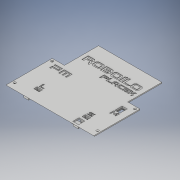
# Autodesk Inventor part: dach2
Saved by Autodesk Inventor 2019 (Build 230136000, 136)
## iProperties
Created: 2019-09-08
Part Number: dach2
Material: Generic
Document SubType Name: Modeling
Designer: Michal
Density: 1 g/cm^3
Appearance: Default
Author: Michal
Autodesk Inventor part; units mm, degrees
ref_plane "YZ Plane" through (0, 0, 0) normal (1, 0, 0) x (0, 1, 0)
ref_plane "XZ Plane" through (0, 0, 0) normal (0, 1, 0) x (-1, 0, 0)
ref_plane "XY Plane" through (0, 0, 0) normal (0, 0, 1) x (1, 0, 0)
sketch "Sketch1" plane through (0, 0, 0) normal (0, 1, 0) x (-1, 0, 0)
  line L0 (0, 0) -> (180, 0)
  line L1 (180, 0) -> (180, -95)
  line L2 (0, 0) -> (0, -95)
  line L3 (180, -95) -> (155, -95)
  line L4 (0, -95) -> (25, -95)
  line L5 (25, -95) -> (25, -165)
  line L6 (155, -95) -> (155, -165)
  line L7 (155, -165) -> (25, -165)
  dimension "d0" = 180
  dimension "d1" = 95
  dimension "d4" = 95
  dimension "d35" = 25
  dimension "d36" = 25
  constraints: 16 end point, 4 horizontal, 2 perpendicular, 2 vertical
  measures "d0" distance of L0.start L0.end
  measures "d1" distance of L0.end L1.end
  measures "d4" distance of L0.start L2.end
  measures "d35" distance of L1.end L3.end
  measures "d36" distance of L2.end L4.end
extrude "Extrusion1" add sketch "Sketch1" along normal blind 2
sketch "Sketch3" plane through (-155, 0, -165) normal (-1, 0, 0) x (0, 0, 1)
  line L0 (70, 2) -> (0, 2) projected
  line L1 (0, 2) -> (28, 2)
  line L2 (28, 2) -> (28, -13)
  circle A0 centre (28, -13) radius 12.5
  point P0 (165, 0)
  dimension "d46" = 28
  dimension "d47" = 15
  dimension "d48" = 25
  constraints: 4 end point, 1 centre point, 1 coincident, 1 perpendicular, 1 point on line
  measures "d46" distance of L0.end L1.end
  measures "d47" distance of L1.end L2.end
  measures "d48" diameter of A0
extrude "Extrusion3" cut sketch "Sketch3" against normal blind 130
chamfer "Chamfer1" distance 2 angle 45 1 edges at (-90, 0, 0)
sketch "Sketch22" plane through (0, 0, 0) normal (0, -1, 0) x (1, 0, 0)
  line L0 (0, -95.1062) -> (-10, -95.1062)
  line L1 (-10, -95.1062) -> (-10, -85.1062)
  line L2 (-10, -85.1062) -> (0, -85.1062)
  line L3 (-180, -85.1062) -> (-180, -95.1062)
  line L4 (0, -95) -> (0, -2) projected
  line L5 (0, -2) -> (-34, -2)
  line L6 (-180, -2) -> (0, -2) projected
  line L7 (-34, -2) -> (-44, -2)
  line L8 (-10, -85.1062) -> (-10, -46.6062)
  line L9 (-10, -46.6062) -> (-34, -46.6062)
  line L10 (-34, -46.6062) -> (-34, -2)
  line L11 (-10, -85.1062) -> (-25, -85.1062)
  line L12 (-25, -95) -> (-25, -165) projected
  line L13 (-44, -2) -> (-44, -46.6062)
  line L14 (-44, -46.6062) -> (-44, -56.6062)
  line L15 (-44, -56.6062) -> (-25, -56.6062)
  line L16 (-25, -56.6062) -> (-25, -85.1062)
  line L17 (-180, -95.1062) -> (-170, -95.1062)
  line L18 (-170, -95.1062) -> (-170, -85.1062)
  line L19 (-170, -85.1062) -> (-180, -85.1062)
  line L20 (-180, -2) -> (-146, -2)
  line L21 (-146, -2) -> (-136, -2)
  line L22 (-170, -85.1062) -> (-170, -46.6062)
  line L23 (-170, -46.6062) -> (-146, -46.6062)
  line L24 (-146, -46.6062) -> (-146, -2)
  line L25 (-170, -85.1062) -> (-155, -85.1062)
  line L26 (-136, -2) -> (-136, -46.6062)
  line L27 (-136, -46.6062) -> (-136, -56.6062)
  line L28 (-136, -56.6062) -> (-155, -56.6062)
  line L29 (-155, -56.6062) -> (-155, -85.1062)
  line L30 (-25, -165) -> (-38.1, -165)
  line L31 (-25, -165) -> (-155, -165) projected
  line L32 (-155, -165) -> (-155, -95) projected
  line L33 (-155, -165) -> (-141.9, -165)
  line L34 (-38.1, -165) -> (-141.9098, -165)
  line L35 (-141.9098, -165) -> (-141.9098, -113)
  line L36 (-141.9098, -113) -> (-38.1, -113)
  line L37 (-38.1, -113) -> (-38.1, -165)
  line L38 (-34, -2) -> (-34, -2.25)
  line L39 (-34, -2.25) -> (-44, -2.25)
  line L40 (-34, -2.25) -> (-34.25, -2.25)
  line L41 (-34.25, -2.25) -> (-34.25, -46.6062)
  line L42 (-34.25, -46.6062) -> (-34.25, -46.8562)
  line L43 (-34.25, -46.8562) -> (-10, -46.8562)
  line L44 (-10, -46.8562) -> (-10.25, -46.8562)
  line L45 (-10.25, -46.8562) -> (-10.25, -85.1062)
  line L46 (-10.25, -85.1062) -> (-10.25, -84.8562)
  line L47 (-10.25, -84.8562) -> (-25, -84.8562)
  line L48 (-146, -2) -> (-146, -2.25)
  line L49 (-146, -2.25) -> (-136, -2.25)
  line L50 (-146, -2.25) -> (-145.75, -2.25)
  line L51 (-145.75, -2.25) -> (-145.75, -46.6062)
  line L52 (-145.75, -46.6062) -> (-145.75, -46.8562)
  line L53 (-145.75, -46.8562) -> (-170, -46.8562)
  line L54 (-170, -46.8562) -> (-169.75, -46.8562)
  line L55 (-169.75, -85.1062) -> (-169.75, -84.8562)
  line L56 (-169.75, -84.8562) -> (-155, -84.8562)
  line L57 (-141.9098, -165) -> (-141.6598, -165)
  line L58 (-155, -165) -> (-25, -165) projected
  line L59 (-141.6598, -165) -> (-141.6598, -113)
  line L60 (-38.1, -113) -> (-38.35, -113)
  line L61 (-38.35, -113) -> (-38.35, -165)
  line L62 (-169.75, -84.8562) -> (-169.75, -46.8562)
  point P0 (0, 0)
  dimension "d215" = 10
  dimension "d216" = 10
  dimension "d217" = 34
  dimension "d218" = 10
  dimension "d219" = 38.5
  dimension "d220" = 10
  dimension "d221" = 13.1
  dimension "d222" = 13.1
  dimension "d223" = 103.8098
  dimension "d224" = 52
  dimension "d234" = 0.25
  dimension "d235" = 0.25
  dimension "d236" = 0.25
  dimension "d237" = 0.25
  dimension "d238" = 0.25
  dimension "d239" = 0.25
  dimension "d240" = 0.25
  dimension "d241" = 0.25
  dimension "d242" = 0.25
  dimension "d243" = 0.25
  dimension "d244" = 0.25
  dimension "d245" = 0.25
  constraints: 112 end point, 28 point on line, 17 perpendicular, 5 parallel, 3 vertical, 2 horizontal, 1 coincident, 4 other
  measures "d215" distance of L2.end L1.end
  measures "d216" distance of L0.end L1.end
  measures "d217" distance of L5.start L5.end
  measures "d218" distance of L5.end L7.end
  measures "d219" distance of L1.end L8.end
  measures "d220" distance of L13.end L14.end
  measures "d221" distance of L12.end L30.end
  measures "d222" distance of L31.end L33.end
  measures "d223" distance of L35.end L36.end
  measures "d224" distance of L34.end L35.end
  measures "d234" distance of L5.end L38.end
  measures "d235" distance of L38.end L40.end
  measures "d236" distance of L41.end L42.end
  measures "d237" distance of L43.end L44.end
  measures "d238" distance of L45.end L46.end
  measures "d239" distance of L20.end L48.end
  measures "d240" distance of L48.end L50.end
  measures "d241" distance of L51.end L52.end
  measures "d242" distance of L53.end L54.end
  measures "d243" distance of L55.start L55.end
  measures "d244" distance of L34.end L57.end
  measures "d245" distance of L36.end L60.end
extrude "Extrusion24" add sketch "Sketch22" along normal blind 4 contours L45 L47 L16 L15 L14 L13 L39 L41 L42 L43 | L53 L52 L51 L49 L26 L27 L28 L29 L56 L62 | L31 L61 L36 L37 | L31 L59 L36 L61 | L31 L35 L36 L59
sketch "Sketch7" plane through (0, 2, 0) normal (0, 1, 0) x (1, 0, 0)
  line L0 (-155, 95) -> (-180, 95) projected
  line L1 (-180, 95) -> (-175, 95)
  line L2 (-175, 95) -> (-175, 90)
  line L3 (-175, 90) -> (-180, 90)
  line L4 (-180, 90) -> (-180, 95)
  line L5 (0, 95) -> (-25, 95) projected
  line L6 (0, 95) -> (-5, 95)
  line L7 (-5, 95) -> (-5, 90)
  line L8 (-5, 90) -> (0, 90)
  line L9 (0, 90) -> (0, 95)
  line L10 (-5, 90) -> (-5, 13)
  line L11 (-175, 90) -> (-175, 13)
  point P0 (0, 0)
  dimension "d80" = 5
  dimension "d81" = 5
  dimension "d82" = 5
  dimension "d83" = 77
  constraints: 20 end point, 4 parallel, 2 horizontal, 2 perpendicular, 2 vertical, 1 point on line
  measures "d80" distance of L2.end L3.end
  measures "d81" distance of L1.end L2.end
  measures "d82" distance of L8.end L7.end
  measures "d83" distance of L7.end L10.end
hole "Hole1" at (-175, 2, -90) at (-5, 2, -90) at (-5, 2, -13) at (-175, 2, -13) direction (0, -1, 0) diameter 2.4638 depth 8.7884 countersink diameter 5 countersink angle 75
sketch "Sketch8" plane through (0, 2, 0) normal (0, 1, 0) x (1, 0, 0)
  line L0 (0, 0) -> (0, 95) projected
  line L1 (0, 95) -> (-13, 95)
  line L2 (-13, 95) -> (-13, 82)
  line L3 (-13, 82) -> (0, 82)
  line L4 (0, 82) -> (0, 95)
  line L5 (-13, 82) -> (-23.5, 82)
  line L6 (-23.5, 82) -> (-23.5, 67)
  line L7 (-23.5, 67) -> (-13, 67)
  line L8 (-13, 67) -> (-13, 82)
  line L9 (-180, 95) -> (-180, 0) projected
  line L10 (-180, 0) -> (0, 0) projected
  line L11 (0, 0) -> (-35, 0)
  line L12 (-35, 0) -> (-35, 4)
  line L13 (-35, 4) -> (0, 4)
  line L14 (0, 4) -> (0, 0)
  line L15 (-35, 4) -> (-47, 4)
  line L16 (-47, 4) -> (-47, 17)
  line L17 (-47, 17) -> (-35, 17)
  line L18 (-35, 17) -> (-35, 4)
  line L19 (-35, 17) -> (-35, 22)
  line L20 (-35, 22) -> (-46, 22)
  line L21 (-46, 22) -> (-46, 29)
  line L22 (-46, 29) -> (-35, 29)
  line L23 (-35, 29) -> (-35, 22)
  line L24 (-180, 0) -> (-145, 0)
  line L25 (-145, 0) -> (-145, 22)
  line L26 (-145, 22) -> (-180, 22)
  line L27 (-180, 22) -> (-180, 0)
  line L28 (-145, 22) -> (-134, 22)
  line L29 (-134, 22) -> (-134, 29)
  line L30 (-134, 29) -> (-145, 29)
  line L31 (-145, 29) -> (-145, 22)
  dimension "d91" = 13
  dimension "d92" = 13
  dimension "d93" = 10.5
  dimension "d94" = 15
  dimension "d128" = 35
  dimension "d129" = 4
  dimension "d130" = 12
  dimension "d131" = 13
  dimension "d141" = 5
  dimension "d142" = 11
  dimension "d143" = 7
  dimension "d158" = 35
  dimension "d159" = 22
  dimension "d160" = 11
  dimension "d161" = 7
  constraints: 58 end point, 14 parallel, 7 horizontal, 7 perpendicular, 1 vertical
  measures "d91" distance of L3.end L2.end
  measures "d92" distance of L2.end L1.end
  measures "d93" distance of L7.end L6.end
  measures "d94" distance of L6.end L5.end
  measures "d128" distance of L12.end L13.end
  measures "d129" distance of L11.end L12.end
  measures "d130" distance of L16.end L17.end
  measures "d131" distance of L15.end L16.end
  measures "d141" distance of L17.end L19.end
  measures "d142" distance of L21.end L22.end
  measures "d143" distance of L20.end L21.end
  measures "d158" distance of L26.end L25.end
  measures "d159" distance of L25.end L24.end
  measures "d160" distance of L30.end L29.end
  measures "d161" distance of L29.end L28.end
extrude "Extrusion7" cut sketch "Sketch8" against normal blind 7 contours L15 L16 L17 L18 | L8 L7 L6 L5 | L31 L30 L29 L28 | L20 L21 L22 L23
sketch "Sketch9" plane through (0, 0, 0) normal (0, -1, 0) x (1, 0, 0)
  line L0 (-13, -67) -> (-23.5, -67) projected
  line L1 (-23.5, -67) -> (-23.5, -82) projected
  line L2 (-13, -67) -> (-23.5, -67)
  line L3 (-23.5, -67) -> (-23.5, -82)
  line L4 (-23.5, -82) -> (-13, -82)
  line L5 (-13, -82) -> (-13, -67)
  line L6 (-23.5, -82) -> (-13, -82) projected
  line L7 (-11, -65) -> (-25.5, -65)
  line L8 (-25.5, -65) -> (-25.5, -84)
  line L9 (-25.5, -84) -> (-11, -84)
  line L10 (-11, -84) -> (-11, -65)
  line L11 (-11, -84) -> (-11, -65)
  line L12 (-10, -85) -> (-10, -84)
  line L13 (-180, -2) -> (-180, -95) projected
  point P0 (0, 0)
  point P1 (-155, -165)
  dimension "d181" = 1
  constraints: 20 end point, 4 parallel, 2 horizontal, 2 perpendicular
  measures "d181" distance of L12.end L11.start
extrude "Extrusion8" add sketch "Sketch9" along normal blind 3
sketch "Sketch10" plane through (-13, 2, -82) normal (-1, 0, 0) x (0, 0, 1)
  line L0 (0, 0) -> (15, 0) projected
  line L1 (0, 0) -> (0, -3)
  line L2 (0, 0) -> (0, -6) projected
  line L3 (15, 0) -> (15, -6) projected
  line L4 (0, -3) -> (15, -3)
  line L5 (15, -3) -> (15, -5)
  line L6 (15, -5) -> (0, -5)
  line L7 (0, -5) -> (0, -3)
  point P0 (82, -2)
  point P1 (0, -5)
  point P2 (0, -2)
  point P3 (15, -2)
  dimension "d103" = 3
  constraints: 10 end point, 2 parallel, 1 horizontal, 1 midpoint, 1 perpendicular
  measures "d103" distance of L0.start L1.end
extrude "Extrusion9" add sketch "Sketch10" along normal blind 1 contours L4 L3 L6 L2
sketch "Sketch11" plane through (-23.5, 2, -67) normal (1, 0, 0) x (0, 0, -1)
  line L0 (15, 0) -> (15, -3) projected
  line L1 (15, 0) -> (15, -3)
  line L2 (0, -3) -> (15, -3) projected
  line L3 (15, -5) -> (0, -5) projected
  line L4 (15, -3) -> (0, -3)
  line L5 (0, -3) -> (0, -5)
  line L6 (0, -5) -> (15, -5)
  line L7 (15, -5) -> (15, -3)
  point P0 (-67, -2)
  point P1 (15, -2)
  constraints: 10 end point, 2 parallel, 1 horizontal, 1 perpendicular, 1 vertical
extrude "Extrusion10" add sketch "Sketch11" along normal blind 1
sketch "Sketch12" plane through (-23.5, 2, -82) normal (0, 0, 1) x (1, 0, 0)
  line L0 (9.5, -3) -> (9.5, -5) projected
  line L1 (1, -3) -> (0, -3) projected
  line L2 (9.5, -5) -> (1, -5)
  line L3 (1, -5) -> (1, -3)
  line L4 (1, -3) -> (9.5, -3)
  line L5 (9.5, -3) -> (9.5, -5)
  point P0 (23.5, -2)
  constraints: 8 end point, 2 parallel, 1 horizontal, 1 perpendicular
extrude "Extrusion11" add sketch "Sketch12" along normal blind 1.3
sketch "Sketch13" plane through (-13, 2, -67) normal (0, 0, -1) x (-1, 0, 0)
  line L0 (0, -3) -> (1, -3) projected
  line L1 (12, -5) -> (12.5, -5) projected
  line L2 (0, -3) -> (10.5024, -3)
  line L3 (10.5024, -3) -> (10.5024, -5)
  line L4 (10.5024, -5) -> (0, -5)
  line L5 (0, -5) -> (0, -3)
  point P0 (-13, -2)
  point P1 (-2, -5)
  point P2 (-3, -5)
  constraints: 8 end point, 2 parallel, 1 horizontal, 1 perpendicular, 1 point on line
extrude "Extrusion12" add sketch "Sketch13" along normal blind 1.3
sketch "Sketch14" plane through (0, -3, 0) normal (0, -1, 0) x (1, 0, 0)
  line L0 (-22.5, -68.3) -> (-22.5, -67)
  line L1 (-13, -67) -> (-23.5, -67) projected
  line L2 (-22.5, -67) -> (-14, -67)
  line L3 (-22.5, -68.3) -> (-14, -68.3) projected
  line L4 (-14, -67) -> (-14, -68.3)
  line L5 (-14, -68.3) -> (-22.5, -68.3)
  line L6 (-22.5, -80.7) -> (-22.5, -68.3) projected
  line L7 (-22.5, -80.7) -> (-22.5, -82)
  line L8 (-23.5, -82) -> (-13, -82) projected
  line L9 (-14, -80.7) -> (-22.5, -80.7) projected
  line L10 (-22.5, -80.7) -> (-14, -80.7)
  line L11 (-14, -80.7) -> (-14, -82)
  line L12 (-14, -82) -> (-22.5, -82)
  point P0 (0, 0)
  constraints: 16 end point, 3 perpendicular, 2 collinear, 2 point on line, 2 vertical, 1 horizontal
extrude "Extrusion13" cut sketch "Sketch14" against normal blind 1
sketch "Sketch17" plane through (0, 0, 0) normal (0, -1, 0) x (1, 0, 0)
  line L0 (-47, -4) -> (-44, -4) projected
  line L1 (-44, -17) -> (-47, -17) projected
  line L2 (-35, -4) -> (-47, -4)
  line L3 (-47, -4) -> (-47, -17)
  line L4 (-47, -17) -> (-35, -17)
  line L5 (-35, -17) -> (-35, -4)
  line L6 (-34, -4) -> (-34, -3)
  line L7 (-34, -3) -> (-35, -3)
  line L8 (-48, -17) -> (-48, -18)
  line L9 (-48, -18) -> (-47, -18)
  line L10 (-48, -18) -> (-34, -18)
  line L11 (-34, -18) -> (-34, -3)
  line L12 (-34, -3) -> (-48, -3)
  line L13 (-48, -3) -> (-48, -18)
  point P0 (0, 0)
  dimension "d132" = 1
  dimension "d133" = 1
  dimension "d134" = 1
  dimension "d135" = 1
  constraints: 24 end point, 4 parallel, 2 horizontal, 2 perpendicular
  measures "d132" distance of L7.end L6.end
  measures "d133" distance of L6.end L6.start
  measures "d134" distance of L9.end L8.end
  measures "d135" distance of L8.end L8.start
extrude "Extrusion16" add sketch "Sketch17" along normal blind 0.5
sketch "Sketch18" plane through (0, -0.5, 0) normal (0, -1, 0) x (1, 0, 0)
  line L0 (-34, -3) -> (-48, -3) projected
  line L1 (-34, -18) -> (-34, -3) projected
  line L2 (-48, -3) -> (-34, -3)
  line L3 (-34, -3) -> (-34, -13)
  line L4 (-34, -13) -> (-48, -13)
  line L5 (-48, -13) -> (-48, -3)
  point P0 (0, 0)
  point P1 (-44, -3)
  dimension "d138" = 10
  constraints: 8 end point, 2 parallel, 1 horizontal, 1 perpendicular, 1 point on line
  measures "d138" distance of L2.end L3.end
extrude "Extrusion17" add sketch "Sketch18" along normal blind 1
sketch "Sketch19" plane through (0, 0, 0) normal (0, -1, 0) x (1, 0, 0)
  line L0 (-46, -22) -> (-44, -22) projected
  line L1 (-35, -22) -> (-46, -22)
  line L2 (-46, -22) -> (-46, -29)
  line L3 (-46, -29) -> (-35, -29)
  line L4 (-35, -29) -> (-35, -22)
  line L5 (-47, -30) -> (-34, -30)
  line L6 (-34, -30) -> (-34, -21)
  line L7 (-34, -21) -> (-47, -21)
  line L8 (-47, -21) -> (-47, -30)
  line L9 (-134, -22) -> (-145, -22)
  line L10 (-145, -22) -> (-145, -29)
  line L11 (-145, -29) -> (-134, -29)
  line L12 (-134, -29) -> (-134, -22)
  line L13 (-146, -30) -> (-133, -30)
  line L14 (-133, -30) -> (-133, -21)
  line L15 (-133, -21) -> (-146, -21)
  line L16 (-146, -21) -> (-146, -30)
  line L17 (-34, -21) -> (-34.25, -21)
  line L18 (-34.25, -21) -> (-34.25, -30)
  line L19 (-34.25, -30) -> (-34, -30)
  line L20 (-34, -30) -> (-34, -21)
  line L21 (-146, -30) -> (-145.75, -30)
  line L22 (-145.75, -30) -> (-145.75, -21)
  line L23 (-145.75, -21) -> (-146, -21)
  line L24 (-146, -21) -> (-146, -30)
  point P0 (0, 0)
  dimension "d251" = 0.25
  dimension "d252" = 0.25
  constraints: 48 end point, 12 parallel, 6 horizontal, 6 perpendicular, 2 point on line
  measures "d251" distance of L19.end L18.end
  measures "d252" distance of L23.end L22.end
extrude "Extrusion18" add sketch "Sketch19" along normal blind 4
sketch "Sketch20" plane through (0, -4, 0) normal (0, -1, 0) x (1, 0, 0)
  line L0 (-34, -30) -> (-47, -30) projected
  line L1 (-47, -21) -> (-34, -21) projected
  line L2 (-34, -30) -> (-47, -30)
  line L3 (-47, -30) -> (-47, -21)
  line L4 (-47, -21) -> (-34, -21)
  line L5 (-34, -21) -> (-34, -30)
  line L6 (-46, -22) -> (-46, -29) projected
  line L7 (-46, -29) -> (-35, -29) projected
  line L8 (-46, -22) -> (-42, -22)
  line L9 (-42, -22) -> (-42, -29)
  line L10 (-42, -29) -> (-46, -29)
  line L11 (-46, -29) -> (-46, -22)
  line L12 (-35, -22) -> (-46, -22) projected
  line L13 (-35, -29) -> (-39, -29)
  line L14 (-39, -29) -> (-39, -22)
  line L15 (-39, -22) -> (-35, -22)
  line L16 (-35, -22) -> (-35, -29)
  line L17 (-133, -30) -> (-146, -30) projected
  line L18 (-133, -30) -> (-146, -30)
  line L19 (-146, -30) -> (-146, -21)
  line L20 (-146, -21) -> (-133, -21)
  line L21 (-133, -21) -> (-133, -30)
  line L22 (-145, -22) -> (-141, -22)
  line L23 (-141, -22) -> (-141, -29)
  line L24 (-141, -29) -> (-145, -29)
  line L25 (-145, -29) -> (-145, -22)
  line L26 (-134, -29) -> (-138, -29)
  line L27 (-138, -29) -> (-138, -22)
  line L28 (-138, -22) -> (-134, -22)
  line L29 (-134, -22) -> (-134, -29)
  line L30 (-34, -30) -> (-34.25, -30)
  line L31 (-34.25, -30) -> (-34.25, -21)
  line L32 (-34.25, -21) -> (-34, -21)
  line L33 (-34, -21) -> (-34, -30)
  line L34 (-146, -30) -> (-133, -30) projected
  line L35 (-133, -21) -> (-146, -21) projected
  line L36 (-146, -30) -> (-145.75, -30)
  line L37 (-145.75, -30) -> (-145.75, -21)
  line L38 (-145.75, -21) -> (-146, -21)
  line L39 (-146, -21) -> (-146, -30)
  point P0 (0, 0)
  point P1 (-44, -30)
  point P2 (-44, -21)
  point P3 (-136, -30)
  dimension "d150" = 4
  dimension "d151" = 4
  dimension "d162" = 4
  dimension "d163" = 4
  dimension "d253" = 0.25
  dimension "d254" = 0.25
  constraints: 64 end point, 16 parallel, 8 horizontal, 8 perpendicular, 4 point on line
  measures "d150" distance of L9.end L10.end
  measures "d151" distance of L14.end L15.end
  measures "d162" distance of L23.end L25.start
  measures "d163" distance of L28.start L29.start
  measures "d253" distance of L31.end L32.end
  measures "d254" distance of L38.end L37.end
sketch "Sketch5" plane through (0, 2, 0) normal (0, 1, 0) x (1, 0, 0)
  line L0 (-154.7367, 165.2131) -> (-24.9468, 165.2131) construction
  line L1 (-24.9468, 165.2131) -> (-24.9468, 95.1481) construction
  line L2 (-24.9468, 95.1481) -> (-154.7367, 95.1481) construction
  line L3 (-154.7367, 95.1481) -> (-154.7367, 165.2131) construction
  line L4 (-180, 2) -> (-180, 95) projected
  line L5 (-166.0933, 87.2081) -> (-150.8913, 87.2081)
  line L6 (-150.8913, 87.2081) -> (-150.8913, 78.7451)
  line L7 (-166.0933, 87.2081) -> (-166.0933, 84.5691)
  line L8 (-166.0933, 84.5691) -> (-153.5243, 84.5691)
  line L9 (-153.5243, 84.5691) -> (-153.5243, 81.3771)
  line L10 (-153.5243, 81.3771) -> (-166.0933, 81.3771)
  line L11 (-166.0933, 81.3771) -> (-166.0933, 75.6831)
  line L12 (-166.0933, 75.6831) -> (-163.4573, 75.6831)
  line L13 (-163.4573, 75.6831) -> (-163.4573, 78.7451)
  line L14 (-163.4573, 78.7451) -> (-150.8913, 78.7451)
  line L15 (-150.8913, 87.2081) -> (-147.5843, 87.2081)
  line L16 (-147.5843, 87.2081) -> (-147.5843, 75.6831)
  line L17 (-147.5843, 75.6831) -> (-144.9503, 75.6831)
  line L18 (-144.9503, 75.6831) -> (-144.9503, 84.5691)
  line L19 (-144.9503, 84.5691) -> (-133.8883, 84.5691)
  line L20 (-133.8883, 84.5691) -> (-133.8883, 75.6831)
  line L21 (-133.8883, 75.6831) -> (-131.2543, 75.6831)
  line L22 (-131.2543, 75.6831) -> (-131.2543, 87.2081)
  line L23 (-131.2543, 87.2081) -> (-147.5843, 87.2081)
  line L24 (-144.9503, 84.5691) -> (-140.7343, 84.5691)
  line L25 (-133.8883, 84.5691) -> (-138.1043, 84.5691)
  line L26 (-138.1043, 84.5691) -> (-138.1043, 83.0161)
  line L27 (-138.1043, 83.0161) -> (-140.7343, 83.0161)
  line L28 (-140.7343, 83.0161) -> (-140.7343, 75.6831)
  line L29 (-140.7343, 75.6831) -> (-138.1043, 75.6831)
  line L30 (-138.1043, 75.6831) -> (-138.1043, 83.0161)
  line L31 (-97.4333, 120.7168) -> (-29.5125, 120.7168) construction
  line L32 (-29.5125, 120.7168) -> (-29.5125, 109.0375) construction
  line L33 (-29.5125, 109.0375) -> (-97.4333, 109.0375) construction
  line L34 (-97.4333, 109.0375) -> (-97.4333, 120.7168) construction
  line L35 (-143.5128, 40.691) -> (-134.453, 40.691) construction
  line L36 (-134.453, 40.691) -> (-134.453, 31.7717) construction
  line L37 (-134.453, 31.7717) -> (-143.5128, 31.7717) construction
  line L38 (-143.5128, 31.7717) -> (-143.5128, 40.691) construction
  line L39 (-45.8219, 39.1059) -> (-34.3434, 39.1059) construction
  line L40 (-34.3434, 39.1059) -> (-34.3434, 31.5278) construction
  line L41 (-34.3434, 31.5278) -> (-45.8219, 31.5278) construction
  line L42 (-45.8219, 31.5278) -> (-45.8219, 39.1059) construction
  line L43 (-23.8076, 65.0882) -> (-10.783, 65.0882) construction
  line L44 (-10.783, 65.0882) -> (-10.783, 56.1982) construction
  line L45 (-10.783, 56.1982) -> (-23.8076, 56.1982) construction
  line L46 (-23.8076, 56.1982) -> (-23.8076, 65.0882) construction
  line L47 (-131.1694, 121.4211) -> (-135.0949, 123.67)
  line L48 (-135.0949, 123.67) -> (-135.0949, 126.8525)
  line L49 (-135.0949, 126.8525) -> (-136.2896, 128.0171)
  line L50 (-136.2896, 128.0171) -> (-143.7891, 128.0171)
  line L51 (-143.7891, 128.0171) -> (-143.7891, 123.67)
  line L52 (-143.7891, 123.67) -> (-147.7146, 123.67)
  line L53 (-147.7146, 123.67) -> (-147.7146, 136.6611)
  line L54 (-147.7146, 136.6611) -> (-134.1311, 136.6611)
  line L55 (-134.1311, 136.6611) -> (-131.1694, 132.6754)
  line L56 (-131.1694, 132.6754) -> (-133.4183, 129.6535)
  line L57 (-133.4183, 129.6535) -> (-131.1694, 127.3946)
  line L58 (-131.1694, 127.3946) -> (-131.1694, 121.4211)
  line L59 (-135.2053, 132.4044) -> (-136.2494, 133.7697)
  line L60 (-136.2494, 133.7697) -> (-143.7891, 133.7697)
  line L61 (-143.7891, 133.7697) -> (-143.7891, 130.9687)
  line L62 (-143.7891, 130.9687) -> (-136.2595, 130.9687)
  line L63 (-136.2595, 130.9687) -> (-135.2053, 132.4044)
  line L64 (-112.1947, 126.6216) -> (-115.1464, 123.67)
  line L65 (-115.1464, 123.67) -> (-125.989, 123.67)
  line L66 (-125.989, 123.67) -> (-128.9407, 126.6216)
  line L67 (-128.9407, 126.6216) -> (-128.9407, 133.7095)
  line L68 (-128.9407, 133.7095) -> (-125.989, 136.6611)
  line L69 (-125.989, 136.6611) -> (-115.1464, 136.6611)
  line L70 (-115.1464, 136.6611) -> (-112.1947, 133.7095)
  line L71 (-112.1947, 133.7095) -> (-112.1947, 126.6216)
  line L72 (-116.1202, 126.5614) -> (-116.1202, 133.7697)
  line L73 (-116.1202, 133.7697) -> (-125.0152, 133.7697)
  line L74 (-125.0152, 133.7697) -> (-125.0152, 126.5614)
  line L75 (-125.0152, 126.5614) -> (-116.1202, 126.5614)
  line L76 (-93.3807, 127.6456) -> (-96.3323, 123.6499)
  line L77 (-96.3323, 123.6499) -> (-110.0965, 123.6499)
  line L78 (-110.0965, 123.6499) -> (-110.0965, 136.6611)
  line L79 (-110.0965, 136.6611) -> (-96.3323, 136.6611)
  line L80 (-96.3323, 136.6611) -> (-93.3807, 132.6654)
  line L81 (-93.3807, 132.6654) -> (-95.2279, 130.1555)
  line L82 (-95.2279, 130.1555) -> (-93.3807, 127.6456)
  line L83 (-97.6776, 127.6456) -> (-98.6313, 128.8303)
  line L84 (-98.6313, 128.8303) -> (-106.171, 128.8303)
  line L85 (-106.171, 128.8303) -> (-106.171, 126.5614)
  line L86 (-106.171, 126.5614) -> (-98.6313, 126.5614)
  line L87 (-98.6313, 126.5614) -> (-97.6776, 127.6456)
  line L88 (-97.6776, 132.6654) -> (-98.6313, 133.7497)
  line L89 (-98.6313, 133.7497) -> (-106.171, 133.7497)
  line L90 (-106.171, 133.7497) -> (-106.171, 131.4807)
  line L91 (-106.171, 131.4807) -> (-98.6313, 131.4807)
  line L92 (-98.6313, 131.4807) -> (-97.6776, 132.6654)
  line L93 (-74.5766, 126.6216) -> (-77.5283, 123.67)
  line L94 (-77.5283, 123.67) -> (-88.3709, 123.67)
  line L95 (-88.3709, 123.67) -> (-91.3226, 126.6216)
  line L96 (-91.3226, 126.6216) -> (-91.3226, 133.7095)
  line L97 (-91.3226, 133.7095) -> (-88.3709, 136.6611)
  line L98 (-88.3709, 136.6611) -> (-77.5283, 136.6611)
  line L99 (-77.5283, 136.6611) -> (-74.5766, 133.7095)
  line L100 (-74.5766, 133.7095) -> (-74.5766, 126.6216)
  line L101 (-78.5021, 126.5614) -> (-78.5021, 133.7697)
  line L102 (-78.5021, 133.7697) -> (-87.3971, 133.7697)
  line L103 (-87.3971, 133.7697) -> (-87.3971, 126.5614)
  line L104 (-87.3971, 126.5614) -> (-78.5021, 126.5614)
  line L105 (-68.5529, 123.6499) -> (-72.4784, 123.67)
  line L106 (-72.4784, 123.67) -> (-72.4784, 136.6712)
  line L107 (-72.4784, 136.6712) -> (-68.5529, 138.9401)
  line L108 (-68.5529, 138.9401) -> (-68.5529, 123.6499)
  line L109 (-51.2347, 126.5614) -> (-54.1462, 123.6499)
  line L110 (-54.1462, 123.6499) -> (-66.3241, 123.6499)
  line L111 (-66.3241, 123.6499) -> (-66.3241, 136.6712)
  line L112 (-66.3241, 136.6712) -> (-62.3987, 138.9401)
  line L113 (-62.3987, 138.9401) -> (-62.3987, 126.5614)
  line L114 (-62.3987, 126.5614) -> (-51.2347, 126.5614)
  line L115 (-34.0471, 126.6216) -> (-36.9987, 123.67)
  line L116 (-36.9987, 123.67) -> (-47.8414, 123.67)
  line L117 (-47.8414, 123.67) -> (-50.793, 126.6216)
  line L118 (-50.793, 126.6216) -> (-50.793, 133.7095)
  line L119 (-50.793, 133.7095) -> (-47.8414, 136.6611)
  line L120 (-47.8414, 136.6611) -> (-36.9987, 136.6611)
  line L121 (-36.9987, 136.6611) -> (-34.0471, 133.7095)
  line L122 (-34.0471, 133.7095) -> (-34.0471, 126.6216)
  line L123 (-37.9725, 126.5614) -> (-37.9725, 133.7697)
  line L124 (-37.9725, 133.7697) -> (-46.8675, 133.7697)
  line L125 (-46.8675, 133.7697) -> (-46.8675, 126.5614)
  line L126 (-46.8675, 126.5614) -> (-37.9725, 126.5614)
  line L127 (-86.3965, 116.5403) -> (-88.6922, 113.4348)
  line L128 (-88.6922, 113.4348) -> (-94.8096, 113.4348)
  line L129 (-94.8096, 113.4348) -> (-94.8096, 110.5367)
  line L130 (-94.8096, 110.5367) -> (-97.4266, 109.0375)
  line L131 (-97.4266, 109.0375) -> (-97.4266, 119.1975)
  line L132 (-97.4266, 119.1975) -> (-88.3709, 119.1975)
  line L133 (-88.3709, 119.1975) -> (-86.3965, 116.5403)
  line L134 (-89.0938, 116.3596) -> (-89.7831, 117.2699)
  line L135 (-89.7831, 117.2699) -> (-94.8096, 117.2699)
  line L136 (-94.8096, 117.2699) -> (-94.8096, 115.4025)
  line L137 (-94.8096, 115.4025) -> (-89.7831, 115.4025)
  line L138 (-89.7831, 115.4025) -> (-89.0938, 116.3596)
  line L139 (-75.4802, 112.4643) -> (-77.4211, 110.5233)
  line L140 (-77.4211, 110.5233) -> (-85.5398, 110.5233)
  line L141 (-85.5398, 110.5233) -> (-85.5398, 119.2042)
  line L142 (-85.5398, 119.2042) -> (-82.9228, 120.7168)
  line L143 (-82.9228, 120.7168) -> (-82.9228, 112.4643)
  line L144 (-82.9228, 112.4643) -> (-75.4802, 112.4643)
  line L145 (-64.6709, 109.0375) -> (-67.3013, 110.5233)
  line L146 (-67.3013, 110.5233) -> (-67.3013, 113.0198)
  line L147 (-67.3013, 113.0198) -> (-72.5687, 113.0198)
  line L148 (-72.5687, 113.0198) -> (-72.5687, 110.5233)
  line L149 (-72.5687, 110.5233) -> (-75.1857, 110.5367)
  line L150 (-75.1857, 110.5367) -> (-75.1857, 117.2565)
  line L151 (-75.1857, 117.2565) -> (-73.2179, 119.1975)
  line L152 (-73.2179, 119.1975) -> (-66.6387, 119.1975)
  line L153 (-66.6387, 119.1975) -> (-64.6709, 117.2565)
  line L154 (-64.6709, 117.2565) -> (-64.6709, 109.0375)
  line L155 (-67.3013, 114.934) -> (-67.3013, 117.2565)
  line L156 (-67.3013, 117.2565) -> (-72.5687, 117.2565)
  line L157 (-72.5687, 117.2565) -> (-72.5687, 114.934)
  line L158 (-72.5687, 114.934) -> (-67.3013, 114.934)
  line L159 (-52.7908, 119.1975) -> (-54.7184, 117.2565)
  line L160 (-54.7184, 117.2565) -> (-60.5414, 117.2565)
  line L161 (-60.5414, 117.2565) -> (-60.5414, 112.4643)
  line L162 (-60.5414, 112.4643) -> (-53.0987, 112.4643)
  line L163 (-53.0987, 112.4643) -> (-55.0397, 110.5233)
  line L164 (-55.0397, 110.5233) -> (-61.1906, 110.5233)
  line L165 (-61.1906, 110.5233) -> (-63.1583, 112.4643)
  line L166 (-63.1583, 112.4643) -> (-63.1583, 117.2163)
  line L167 (-63.1583, 117.2163) -> (-61.1906, 119.1975)
  line L168 (-61.1906, 119.1975) -> (-52.7908, 119.1975)
  line L169 (-41.8344, 119.1975) -> (-43.762, 117.2565)
  line L170 (-43.762, 117.2565) -> (-49.5849, 117.2565)
  line L171 (-49.5849, 117.2565) -> (-49.5849, 115.7439)
  line L172 (-49.5849, 115.7439) -> (-43.0994, 115.7439)
  line L173 (-43.0994, 115.7439) -> (-44.8663, 113.9769)
  line L174 (-44.8663, 113.9769) -> (-49.5849, 113.9769)
  line L175 (-49.5849, 113.9769) -> (-49.5849, 112.4643)
  line L176 (-49.5849, 112.4643) -> (-42.1423, 112.4643)
  line L177 (-42.1423, 112.4643) -> (-44.0832, 110.5233)
  line L178 (-44.0832, 110.5233) -> (-52.2019, 110.5233)
  line L179 (-52.2019, 110.5233) -> (-52.2019, 119.1975)
  line L180 (-52.2019, 119.1975) -> (-41.8344, 119.1975)
  line L181 (-30.7507, 119.1975) -> (-34.0504, 116.0451)
  line L182 (-34.0504, 116.0451) -> (-31.0251, 113.0198)
  line L183 (-31.0251, 113.0198) -> (-31.0251, 110.5233)
  line L184 (-31.0251, 110.5233) -> (-33.6421, 109.0375)
  line L185 (-33.6421, 109.0375) -> (-33.6421, 112.6383)
  line L186 (-33.6421, 112.6383) -> (-35.5764, 114.5726)
  line L187 (-35.5764, 114.5726) -> (-38.3607, 111.9556)
  line L188 (-38.3607, 111.9556) -> (-38.3607, 110.5233)
  line L189 (-38.3607, 110.5233) -> (-40.9777, 110.5367)
  line L190 (-40.9777, 110.5367) -> (-40.9777, 119.1975)
  line L191 (-40.9777, 119.1975) -> (-38.3607, 119.1975)
  line L192 (-38.3607, 119.1975) -> (-38.3607, 114.9474)
  line L193 (-38.3607, 114.9474) -> (-33.8429, 119.1975)
  line L194 (-33.8429, 119.1975) -> (-30.7507, 119.1975)
  line L195 (-134.7048, 33.47) -> (-136.4032, 31.7717)
  line L196 (-136.4032, 31.7717) -> (-143.507, 31.7717)
  line L197 (-143.507, 31.7717) -> (-143.507, 39.3674)
  line L198 (-143.507, 39.3674) -> (-141.2171, 40.691)
  line L199 (-141.2171, 40.691) -> (-141.2171, 33.47)
  line L200 (-141.2171, 33.47) -> (-134.7048, 33.47)
  line L201 (-35.2921, 33.8586) -> (-37.0139, 31.5278)
  line L202 (-37.0139, 31.5278) -> (-45.8161, 31.5278)
  line L203 (-45.8161, 31.5278) -> (-44.1294, 33.2144)
  line L204 (-44.1294, 33.2144) -> (-38.355, 33.2144)
  line L205 (-38.355, 33.2144) -> (-37.8162, 33.8586)
  line L206 (-37.8162, 33.8586) -> (-38.3492, 34.538)
  line L207 (-38.3492, 34.538) -> (-44.1411, 34.538)
  line L208 (-44.1411, 34.538) -> (-45.8161, 36.7751)
  line L209 (-45.8161, 36.7751) -> (-44.0943, 39.1059)
  line L210 (-44.0943, 39.1059) -> (-35.2921, 39.1059)
  line L211 (-35.2921, 39.1059) -> (-36.9905, 37.4193)
  line L212 (-36.9905, 37.4193) -> (-42.7532, 37.4193)
  line L213 (-42.7532, 37.4193) -> (-43.3095, 36.7751)
  line L214 (-43.3095, 36.7751) -> (-42.7532, 36.0958)
  line L215 (-42.7532, 36.0958) -> (-36.9612, 36.0958)
  line L216 (-36.9612, 36.0958) -> (-35.2921, 33.8586)
  line L217 (-12.0655, 57.5101) -> (-14.3554, 57.5101)
  line L218 (-14.3554, 57.5101) -> (-14.3554, 62.3592)
  line L219 (-14.3554, 62.3592) -> (-17.2016, 58.4529)
  line L220 (-17.2016, 58.4529) -> (-18.6832, 58.4529)
  line L221 (-18.6832, 58.4529) -> (-21.5119, 62.3592)
  line L222 (-21.5119, 62.3592) -> (-21.5119, 57.5101)
  line L223 (-21.5119, 57.5101) -> (-23.8017, 56.1982)
  line L224 (-23.8017, 56.1982) -> (-23.8017, 65.0882)
  line L225 (-23.8017, 65.0882) -> (-21.2132, 65.0882)
  line L226 (-21.2132, 65.0882) -> (-17.9336, 60.5788)
  line L227 (-17.9336, 60.5788) -> (-14.6658, 65.0882)
  line L228 (-14.6658, 65.0882) -> (-12.0655, 65.0882)
  line L229 (-12.0655, 65.0882) -> (-12.0655, 57.5101)
  point P0 (0, 0)
  dimension "d166" = 15.202
  dimension "d167" = 8.463
  dimension "d168" = 2.639
  dimension "d169" = 12.569
  dimension "d170" = 3.192
  dimension "d171" = 5.694
  dimension "d172" = 2.636
  dimension "d173" = 3.307
  dimension "d174" = 2.634
  dimension "d175" = 8.886
  dimension "d176" = 11.062
  dimension "d177" = 2.634
  dimension "d178" = 4.216
  dimension "d179" = 4.216
  dimension "d180" = 1.553
  constraints: 52 end point, 15 perpendicular, 7 point on line, 3 horizontal, 3 parallel, 1 vertical, 10 other
  measures "d166" distance of L5.start L5.end
  measures "d167" distance of L5.end L6.end
  measures "d168" distance of L5.start L7.end
  measures "d169" distance of L7.end L8.end
  measures "d170" distance of L8.end L9.end
  measures "d171" distance of L10.end L11.end
  measures "d172" distance of L11.end L12.end
  measures "d173" distance of L5.end L15.end
  measures "d174" distance of L16.end L17.end
  measures "d175" distance of L17.end L18.end
  measures "d176" distance of L18.end L19.end
  measures "d177" distance of L20.end L21.end
  measures "d178" distance of L18.end L24.end
  measures "d179" distance of L19.end L25.end
  measures "d180" distance of L25.end L26.end
extrude "Extrusion6" cut sketch "Sketch5" against normal blind 1
sketch "Sketch23" plane through (0, -1.5, 0) normal (0, -1, 0) x (1, 0, 0)
  line L0 (-44, -4) -> (-35, -4) projected
  line L1 (-48, -13) -> (-34, -13) projected
  line L2 (-44, -4) -> (-35, -4)
  line L3 (-35, -4) -> (-35, -13)
  line L4 (-35, -13) -> (-44, -13)
  line L5 (-44, -13) -> (-44, -4)
  point P0 (0, 0)
  constraints: 8 end point, 2 parallel, 1 horizontal, 1 perpendicular
extrude "Extrusion22" add sketch "Sketch23" along normal blind 2.5
sketch "Sketch24" plane through (-155, 0, -165) normal (-1, 0, 0) x (0, 0, 1)
  line L0 (0, 2) -> (70, 2) projected
  line L1 (0, 2) -> (28, 2)
  line L2 (28, 2) -> (28, -13)
  circle A0 centre (28, -13) radius 12.75
  point P0 (165, 0)
  dimension "d229" = 28
  dimension "d230" = 15
  dimension "d248" = 25.5
  constraints: 4 end point, 1 centre point, 1 coincident, 1 perpendicular, 1 point on line
  measures "d229" distance of L0.start L1.end
  measures "d230" distance of L1.end L2.end
  measures "d248" diameter of A0
extrude "Extrusion23" cut sketch "Sketch24" against normal blind 130
extrude "Extrusion25" add sketch "Sketch20" along normal blind 4 contours L0 L3 L1 L31 | L12 L14 L7 L9 | L17 L37 L20 L21
move faces "Move1" translate (-0.25, 0, 0) faces at (-34, -0.6667, -6.3333)
move faces "Move2" translate (-0.25, 0, 0) faces at (-34, -1.3333, -24)
move faces "Move3" translate (0.25, 0, 0) faces at (-146, -1.3333, -27)
body "Solid1"
